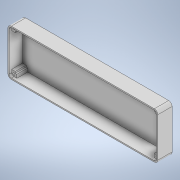
# Autodesk Inventor part: Case Full
Saved by Autodesk Inventor 2020 (Build 240168000, 168)
## iProperties
Created: 2021-04-14
Part Number: Case Full
Material: Generic
Document SubType Name: Modeling
Designer: user
Density: 1 g/cm^3
Appearance: Default
Author: user
Autodesk Inventor part; units mm, degrees
ref_plane "YZ Plane" through (0, 0, 0) normal (1, 0, 0) x (0, 1, 0)
ref_plane "XZ Plane" through (0, 0, 0) normal (0, 1, 0) x (-1, 0, 0)
ref_plane "XY Plane" through (0, 0, 0) normal (0, 0, 1) x (1, 0, 0)
sketch "Sketch1" plane through (0, 0, 0) normal (0, 0, 1) x (1, 0, 0)
  line L0 (5, 0) -> (336, 0)
  line L1 (341, 5) -> (341, 96)
  line L2 (336, 101) -> (5, 101)
  line L3 (0, 96) -> (0, 5)
  arc A0 (5, 101) -> (0, 96) centre (5, 96) ccw
  arc A1 (0, 5) -> (5, 0) centre (5, 5) ccw
  arc A2 (341, 96) -> (336, 101) centre (336, 96) ccw
  arc A3 (336, 0) -> (341, 5) centre (336, 5) ccw
  line L4 (5, 101.2) -> (336, 101.2)
  arc A4 (341.2, 96) -> (336, 101.2) centre (336, 96) ccw
  line L5 (341.2, 96) -> (341.2, 5)
  arc A5 (336, -0.2) -> (341.2, 5) centre (336, 5) ccw
  line L6 (336, -0.2) -> (5, -0.2)
  arc A6 (-0.2, 5) -> (5, -0.2) centre (5, 5) ccw
  line L7 (-0.2, 5) -> (-0.2, 96)
  arc A7 (5, 101.2) -> (-0.2, 96) centre (5, 96) ccw
  line L8 (5, 104) -> (336, 104)
  arc A8 (344, 96) -> (336, 104) centre (336, 96) ccw
  line L9 (344, 96) -> (344, 5)
  arc A9 (336, -3) -> (344, 5) centre (336, 5) ccw
  line L10 (336, -3) -> (5, -3)
  arc A10 (-3, 5) -> (5, -3) centre (5, 5) ccw
  line L11 (-3, 5) -> (-3, 96)
  arc A11 (5, 104) -> (-3, 96) centre (5, 96) ccw
  point P0 (0, 0)
  point P1 (341, 101)
  point P2 (0, 101)
  dimension "d0" = 341
  dimension "d1" = 101
  dimension "d2" = 5
  dimension "d3" = 0.2
  dimension "d4" = 3
  constraints: 24 end point, 24 point on circle, 12 centre point, 8 tangent, 6 parallel, 6 point on line, 3 equal radius, 3 perpendicular, 1 horizontal, 14 other
  measures "d0" distance of point (0, 101) point (341, 101)
  measures "d1" distance of point (0, 101) point (0, 0)
  measures "d2" radius of A0
  measures "d3" distance between parallel lines of L2 L4
  measures "d4" distance between parallel lines of L2 L8
extrude "Extrusion1" add sketch "Sketch1" along normal blind 2 contours A1 L3 A0 L2 A2 L1 A3 L0 | L4 A4 L5 A5 L6 A6 L7 A7 | L8 A8 L9 A9 L10 A10 L11 A11
sketch "Sketch2" plane through (0, 0, 2) normal (0, 0, 1) x (1, 0, 0)
  line L0 (5, 104) -> (336, 104)
  line L1 (344, 96) -> (344, 5)
  line L2 (336, -3) -> (5, -3)
  line L3 (-3, 5) -> (-3, 96)
  line L4 (344, 5) -> (344, 96) projected
  line L5 (5, -3) -> (336, -3) projected
  arc A0 (5, 104) -> (-3, 96) centre (5, 96) ccw
  arc A1 (-3, 5) -> (5, -3) centre (5, 5) ccw
  arc A2 (336, -3) -> (344, 5) centre (336, 5) ccw
  arc A3 (344, 96) -> (336, 104) centre (336, 96) ccw
  line L6 (336, 101.2) -> (5, 101.2)
  arc A4 (5, 101.2) -> (-0.2, 96) centre (5, 96) ccw
  line L7 (-0.2, 96) -> (-0.2, 5)
  arc A5 (-0.2, 5) -> (5, -0.2) centre (5, 5) ccw
  line L8 (5, -0.2) -> (336, -0.2)
  arc A6 (336, -0.2) -> (341.2, 5) centre (336, 5) ccw
  line L9 (341.2, 5) -> (341.2, 96)
  arc A7 (341.2, 96) -> (336, 101.2) centre (336, 96) ccw
  circle A8 centre (5, 96) radius 2.5
  line L10 (9, 92) -> (332, 92)
  line L11 (332, 92) -> (332, 9)
  line L12 (332, 9) -> (9, 9)
  line L13 (9, 9) -> (9, 92)
  line L14 (-0.2, 89.2) -> (8, 89.2)
  line L15 (8, 89.2) -> (8, 93)
  line L16 (8, 93) -> (11.8, 93)
  line L17 (11.8, 93) -> (11.8, 101.2)
  line L18 (9, 9) -> (332, 92)
  line L19 (170.5, 64.427) -> (170.5, 38.8649)
  line L20 (118.7328, 50.5) -> (212.1169, 50.5)
  circle A9 centre (336, 96) radius 2.5
  line L21 (341.2, 89.2) -> (333, 89.2)
  line L22 (333, 89.2) -> (333, 93)
  line L23 (333, 93) -> (329.2, 93)
  line L24 (329.2, 93) -> (329.2, 101.2)
  circle A10 centre (5, 5) radius 2.5
  line L25 (-0.2, 11.8) -> (8, 11.8)
  line L26 (8, 11.8) -> (8, 8)
  line L27 (8, 8) -> (11.8, 8)
  line L28 (11.8, 8) -> (11.8, -0.2)
  line L29 (329.2, 8) -> (329.2, -0.2)
  line L30 (333, 8) -> (329.2, 8)
  line L31 (333, 11.8) -> (333, 8)
  line L32 (341.2, 11.8) -> (333, 11.8)
  circle A11 centre (336, 5) radius 2.5
  point P0 (0, 0)
  dimension "d7" = 0
  dimension "d8" = 0
  dimension "d9" = 8
  dimension "d10" = 2.8
  dimension "d11" = 5
  dimension "d12" = 5.2
  dimension "d13" = 5.2
  dimension "d19" = 9.2
  dimension "d20" = 9.2
  dimension "d21" = 9.2
  dimension "d22" = 9.2
  dimension "d23" = 1
  dimension "d24" = 1
  dimension "d25" = 12
  dimension "d26" = 12
  constraints: 62 end point, 18 symmetric about line, 16 point on circle, 12 centre point, 8 tangent, 6 parallel, 6 perpendicular, 4 horizontal, 3 equal radius, 2 point on line, 1 vertical, 10 other
  measures "d7" distance between parallel lines of L1 L4
  measures "d8" distance between parallel lines of L2 L5
  measures "d9" radius of A0
  measures "d10" distance between parallel lines of L0 L6
  measures "d11" diameter of A8
  measures "d12" distance from line of A8.centre L6
  measures "d13" distance from line of A8.centre L7
  measures "d19" distance between parallel lines of L10 L6
  measures "d20" distance between parallel lines of L13 L7
  measures "d21" distance between parallel lines of L8 L12
  measures "d22" distance between parallel lines of L9 L11
  measures "d23" distance between parallel lines of L10 L16
  measures "d24" distance between parallel lines of L13 L15
  measures "d25" distance between parallel lines of L6 L14
  measures "d26" distance between parallel lines of L7 L17
extrude "Extrusion2" add sketch "Sketch2" along normal blind 25 contours L0 A3 L1 A2 L2 A1 L3 A0 | A7 L9 L21 L22 L23 L24 L6 | L17 L16 L15 L14 L7 A4 L6 | L9 A6 L8 L29 L30 L31 L32 | L25 L26 L27 L28 L8 A5 L7
sketch "Sketch3" plane through (0, 0, 27) normal (0, 0, 1) x (1, 0, 0)
  line L0 (5, 104) -> (336, 104)
  line L1 (344, 96) -> (344, 5)
  line L2 (336, -3) -> (5, -3)
  line L3 (-3, 5) -> (-3, 96)
  arc A0 (5, 104) -> (-3, 96) centre (5, 96) ccw
  arc A1 (-3, 5) -> (5, -3) centre (5, 5) ccw
  arc A2 (336, -3) -> (344, 5) centre (336, 5) ccw
  arc A3 (344, 96) -> (336, 104) centre (336, 96) ccw
  line L4 (336, 101.2) -> (5, 101.2)
  arc A4 (5, 101.2) -> (-0.2, 96) centre (5, 96) ccw
  line L5 (-0.2, 96) -> (-0.2, 5)
  arc A5 (-0.2, 5) -> (5, -0.2) centre (5, 5) ccw
  line L6 (5, -0.2) -> (336, -0.2)
  arc A6 (336, -0.2) -> (341.2, 5) centre (336, 5) ccw
  line L7 (341.2, 5) -> (341.2, 96)
  arc A7 (341.2, 96) -> (336, 101.2) centre (336, 96) ccw
  point P0 (0, 0)
  dimension "d29" = 8
  dimension "d30" = 2.8
  constraints: 16 end point, 16 point on circle, 8 centre point, 8 tangent, 4 parallel, 3 equal radius, 2 perpendicular, 1 horizontal, 7 other
  measures "d29" radius of A0
  measures "d30" distance between parallel lines of L0 L4
extrude "Extrusion3" add sketch "Sketch3" along normal blind 6
body "Solid1"
